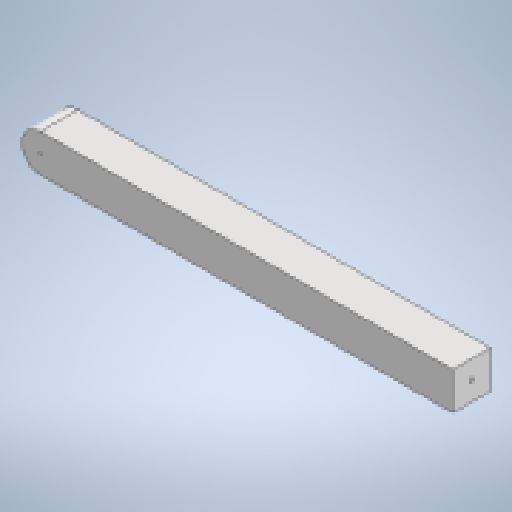
# Autodesk Inventor part: link3
Saved by Autodesk Inventor 2025.4 (Build 294407000, 407)
## iProperties
Created: 2026-03-19
Part Number: link3
Material: Generic
Document SubType Name: Modeling
Designer: dawid
Density: 1 g/cm^3
Appearance: Default
Author: dawid
Autodesk Inventor part; units mm, degrees
ref_plane "YZ Plane" through (0, 0, 0) normal (1, 0, 0) x (0, 1, 0)
ref_plane "XZ Plane" through (0, 0, 0) normal (0, 1, 0) x (-1, 0, 0)
ref_plane "XY Plane" through (0, 0, 0) normal (0, 0, 1) x (1, 0, 0)
sketch "Sketch1" plane through (0, 0, 0) normal (0, 0, 1) x (1, 0, 0)
  circle A0 centre (0, 0) radius 5
  arc A1 (0, 50) -> (0, -50) centre (0, 0) ccw
  line L0 (0, 50) -> (1100, 50)
  line L1 (1100, 50) -> (1100, -50)
  line L2 (1100, -50) -> (0, -50)
  line L3 (0, -50) -> (0, 5)
  dimension "d0" = 10
  dimension "d1" = 100
  dimension "d2" = 1100
  constraints: 8 end point, 2 coincident, 2 parallel, 2 point on circle, 2 tangent, 1 centre point, 1 horizontal, 1 perpendicular, 1 vertical alignment, 2 other
  measures "d1" diameter of A1
  measures "d2" distance of L1.end L2.end
extrude "Extrusion1" add sketch "Sketch1" along normal blind 100
sketch "Sketch2" plane through (1100, -50, 0) normal (1, 0, 0) x (0, 0, -1)
  circle A0 centre (-50, 50) radius 5
  line L0 (0, 0) -> (0, 100) projected
  line L1 (0, 0) -> (-100, 0) projected
  line L2 (-100, 0) -> (-100, 100) projected
  point P0 (0, 50)
  point P1 (0, 50)
  dimension "d5" = 10
  dimension "d6" = 50
  dimension "d7" = 50
  dimension "d8" = 100
  constraints: 1 centre point, 1 midpoint
  measures "d5" diameter of A0
  measures "d6" distance of point (0, 50) A0.centre
  measures "d7" distance from line of L1 A0.centre
  measures "d8" distance between parallel lines of L0 L2
hole "Hole1" at (1100, 0, 50) direction (-1, 0, 0) diameter 10 end through all
equation "\"d6\" = 0.5 * d8"
equation "\"d7\" = d6"
body "Solid1"
